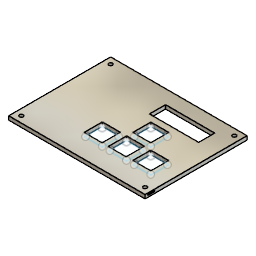
top panel cad file (Autodesk Fusion 360 design; units mm, degrees)
part number: 2026-06-22-21-46-06-251
Autodesk Fusion 360 part; units mm, degrees
sketch "plate-2026-06-22T16_12_38.872Z" plane through (0, 0, 0) normal (0, 1, 0) x (1, 0, 0)
  line L0 (22.075, 16.475) -> (35.075, 16.475)
  line L1 (22.075, 2.475) -> (35.075, 2.475)
  line L2 (21.575, 15.975) -> (21.575, 2.975)
  line L3 (35.575, 15.975) -> (35.575, 2.975)
  arc A0 (22.075, 16.475) -> (21.575, 15.975) centre (22.075, 15.975) ccw
  arc A1 (35.575, 15.975) -> (35.075, 16.475) centre (35.075, 15.975) ccw
  arc A2 (21.575, 2.975) -> (22.075, 2.475) centre (22.075, 2.975) ccw
  arc A3 (35.075, 2.475) -> (35.575, 2.975) centre (35.075, 2.975) ccw
  line L4 (3.025, -2.575) -> (16.025, -2.575)
  line L5 (3.025, -16.575) -> (16.025, -16.575)
  line L6 (2.525, -3.075) -> (2.525, -16.075)
  line L7 (16.525, -3.075) -> (16.525, -16.075)
  arc A4 (3.025, -2.575) -> (2.525, -3.075) centre (3.025, -3.075) ccw
  arc A5 (16.525, -3.075) -> (16.025, -2.575) centre (16.025, -3.075) ccw
  arc A6 (2.525, -16.075) -> (3.025, -16.575) centre (3.025, -16.075) ccw
  arc A7 (16.025, -16.575) -> (16.525, -16.075) centre (16.025, -16.075) ccw
  line L8 (22.075, -2.575) -> (35.075, -2.575)
  line L9 (22.075, -16.575) -> (35.075, -16.575)
  line L10 (21.575, -3.075) -> (21.575, -16.075)
  line L11 (35.575, -3.075) -> (35.575, -16.075)
  arc A8 (22.075, -2.575) -> (21.575, -3.075) centre (22.075, -3.075) ccw
  arc A9 (35.575, -3.075) -> (35.075, -2.575) centre (35.075, -3.075) ccw
  arc A10 (21.575, -16.075) -> (22.075, -16.575) centre (22.075, -16.075) ccw
  arc A11 (35.075, -16.575) -> (35.575, -16.075) centre (35.075, -16.075) ccw
  line L12 (41.125, -2.575) -> (54.125, -2.575)
  line L13 (41.125, -16.575) -> (54.125, -16.575)
  line L14 (40.625, -3.075) -> (40.625, -16.075)
  line L15 (54.625, -3.075) -> (54.625, -16.075)
  arc A12 (41.125, -2.575) -> (40.625, -3.075) centre (41.125, -3.075) ccw
  arc A13 (54.625, -3.075) -> (54.125, -2.575) centre (54.125, -3.075) ccw
  arc A14 (40.625, -16.075) -> (41.125, -16.575) centre (41.125, -16.075) ccw
  arc A15 (54.125, -16.575) -> (54.625, -16.075) centre (54.125, -16.075) ccw
sketch "Sketch2" plane through (0, 0, 0) normal (0, 1, 0) x (1, 0, 0)
  line L0 (-38.375, 44.975) -> (68.625, 44.975)
  line L1 (68.625, 44.975) -> (68.625, -35.025)
  line L2 (68.625, -35.025) -> (-38.375, -35.025)
  line L3 (-38.375, -35.025) -> (-38.375, 44.975)
  line L4 (54.625, -3.075) -> (54.625, -16.075)
  line L5 (22.075, 16.475) -> (35.075, 16.475)
  circle A0 centre (-33.375, -30.025) radius 1.45
  circle A1 centre (63.625, -30.025) radius 1.45
  circle A2 centre (63.625, 39.975) radius 1.45
  circle A3 centre (-33.375, 39.975) radius 1.45
  line L6 (15.625, 33.975) -> (54.125, 33.975)
  line L7 (54.125, 33.975) -> (54.125, 21.475)
  line L8 (54.125, 21.475) -> (15.625, 21.475)
  line L9 (15.625, 21.475) -> (15.625, 33.975)
  dimension "d1" = 107
  dimension "d2" = 80
  dimension "d4" = 14
  dimension "d6" = 28.5
  dimension "d7" = 2.9
  dimension "d8" = 5
  dimension "d9" = 5
  dimension "d10" = 2.9
  dimension "d11" = 5
  dimension "d12" = 5
  dimension "d13" = 2.9
  dimension "d14" = 5
  dimension "d15" = 5
  dimension "d16" = 2.9
  dimension "d17" = 5
  dimension "d18" = 5
  dimension "d19" = 38.5
  dimension "d20" = 12.5
  dimension "d21" = 14.5
  dimension "d22" = 5
  constraint horizontal L0
  constraint vertical L1
  constraint horizontal L2
  constraint vertical L3
  constraint horizontal L6
  constraint vertical L7
  constraint horizontal L8
  constraint vertical L9
  measures "d1" distance of L0.start L0.end
  measures "d2" distance of L0.start L2.end
  measures "d4" distance of L1 L4
  measures "d6" distance of L0 L5
  measures "d7" diameter of A0
  measures "d8" distance of L3 A0.centre
  measures "d9" distance of L2 A0.centre
  measures "d10" diameter of A1
  measures "d11" distance of L1 A1.centre
  measures "d12" distance of L2 A1.centre
  measures "d13" diameter of A2
  measures "d14" distance of L0 A2.centre
  measures "d15" distance of L1 A2.centre
  measures "d16" diameter of A3
  measures "d17" distance of L3 A3.centre
  measures "d18" distance of L0 A3.centre
  measures "d19" distance of L6.start L6.end
  measures "d20" distance of L6.start L8.end
  measures "d21" distance of L1 L7
  measures "d22" distance of L5 L8
sketch "Sketch3" plane through (0, 0, 0) normal (0, 1, 0) x (1, 0, 0)
  line L0 (2.564, -2.4733) -> (16.5959, -2.4733)
  line L1 (16.5959, -2.4733) -> (16.5959, -16.6519)
  line L2 (16.5959, -16.6519) -> (2.564, -16.6519)
  line L3 (2.564, -16.6519) -> (2.564, -2.4733)
  line L4 (21.6806, 16.3989) -> (35.6147, 16.3989)
  line L5 (35.6147, 16.3989) -> (35.6147, 2.367)
  line L6 (35.6147, 2.367) -> (21.6806, 2.367)
  line L7 (21.6806, 2.367) -> (21.6806, 16.3989)
  line L8 (21.5463, -2.4528) -> (35.4907, -2.4528)
  line L9 (35.4907, -2.4528) -> (35.4907, -16.7325)
  line L10 (35.4907, -16.7325) -> (21.5463, -16.7325)
  line L11 (21.5463, -16.7325) -> (21.5463, -2.4528)
  line L12 (40.6624, -2.7115) -> (54.7035, -2.7115)
  line L13 (54.7035, -2.7115) -> (54.7035, -16.5966)
  line L14 (54.7035, -16.5966) -> (40.6624, -16.5966)
  line L15 (40.6624, -16.5966) -> (40.6624, -2.7115)
  constraint horizontal L0
  constraint vertical L1
  constraint horizontal L2
  constraint vertical L3
  constraint horizontal L4
  constraint vertical L5
  constraint horizontal L6
  constraint vertical L7
  constraint horizontal L8
  constraint vertical L9
  constraint horizontal L10
  constraint vertical L11
  constraint horizontal L12
  constraint vertical L13
  constraint horizontal L14
  constraint vertical L15
extrude "Extrude1" add sketch "Sketch2" along normal blind 3
extrude "Extrude2" cut sketch "Sketch3" along normal blind 3
sketch "Sketch4" plane through (68.625, 0, 0) normal (1, 0, 0) x (0, 0, -1)
  line L0 (-35.025, 0) -> (44.975, 0)
  line L1 (44.975, 0) -> (44.975, 3)
  line L2 (44.975, 3) -> (-35.025, 3)
  line L3 (-35.025, 3) -> (-35.025, 0)
  line L4 (-32.9, 0.7) -> (-26.4, 0.7) construction
  line L5 (-26.4, 0.7) -> (-26.4, 2.5) construction
  line L6 (-26.4, 2.5) -> (-32.9, 2.5) construction
  line L7 (-32.9, 2.5) -> (-32.9, 0.7) construction
  dimension "d27" = 1
  text T0 "hackpad" font "Arial" height 1 align left top in box 6.5 x 1.8 at (-32.9, 0.7) x (1, 0) y (0, 1) spacing 1
extrude "Extrude3" add sketch "Sketch4" along normal blind 0.2 text T0
equation "d28 = 'hackpad'"
